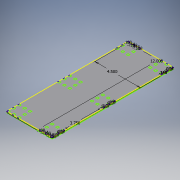
# Autodesk Inventor part: Part1
Saved by Autodesk Inventor 2018 (Build 220112000, 112)
## iProperties
Created: 2018-04-10
Part Number: Part1
Material: Generic
Document SubType Name: Modeling
Designer: Administrator
Density: 1 g/cm^3
Appearance: Default
Author: Administrator
Autodesk Inventor part; units mm, degrees
ref_plane "YZ Plane" through (0, 0, 0) normal (1, 0, 0) x (0, 1, 0)
ref_plane "XZ Plane" through (0, 0, 0) normal (0, 1, 0) x (-1, 0, 0)
ref_plane "XY Plane" through (0, 0, 0) normal (0, 0, 1) x (1, 0, 0)
sketch "Sketch1" plane through (0, 0, 0) normal (0, 1, 0) x (-1, 0, 0)
  line L0 (75.1783, 185.4548) -> (-39.1217, 185.4548)
  line L1 (-39.1217, 185.4548) -> (-39.1217, -119.3452)
  line L2 (-39.1217, -119.3452) -> (75.1783, -119.3452)
  line L3 (75.1783, -119.3452) -> (75.1783, 185.4548)
  point P0 (0, 0)
  dimension "d0" = 304.8
  dimension "d1" = 114.3
  constraints: 8 end point, 2 parallel, 1 horizontal, 1 perpendicular
  measures "d0" distance of L2.end L0.start
  measures "d1" distance of L1.end L2.end
extrude "Extrusion4" add sketch "Sketch1" along normal blind 3
sketch "Sketch11" plane through (0, 3, 0) normal (0, 1, 0) x (1, 0, 0)
  line L0 (39.1217, -185.4548) -> (34.3592, -185.4548)
  line L1 (34.3592, -185.4548) -> (34.3592, -180.6923)
  line L2 (34.3592, -180.6923) -> (39.1217, -180.6923)
  line L3 (39.1217, -180.6923) -> (39.1217, -185.4548)
  line L4 (39.1217, -185.4548) -> (39.1217, 119.3452) projected
  line L5 (39.1217, 119.3452) -> (-75.1783, 119.3452) projected
  line L6 (-75.1783, -185.4548) -> (39.1217, -185.4548) projected
  line L7 (25.628, -185.4548) -> (20.8655, -185.4548)
  line L8 (20.8655, -185.4548) -> (20.8655, -180.6923)
  line L9 (20.8655, -180.6923) -> (25.628, -180.6923)
  line L10 (25.628, -180.6923) -> (25.628, -185.4548)
  line L11 (12.1342, -185.4548) -> (7.3717, -185.4548)
  line L12 (7.3717, -185.4548) -> (7.3717, -180.6923)
  line L13 (7.3717, -180.6923) -> (12.1342, -180.6923)
  line L14 (12.1342, -180.6923) -> (12.1342, -185.4548)
  line L15 (39.1217, -171.961) -> (34.3592, -171.961)
  line L16 (34.3592, -171.961) -> (34.3592, -167.1985)
  line L17 (34.3592, -167.1985) -> (39.1217, -167.1985)
  line L18 (39.1217, -167.1985) -> (39.1217, -171.961)
  line L19 (39.1217, -158.4673) -> (34.3592, -158.4673)
  line L20 (34.3592, -158.4673) -> (34.3592, -153.7048)
  line L21 (34.3592, -153.7048) -> (39.1217, -153.7048)
  line L22 (39.1217, -153.7048) -> (39.1217, -158.4673)
  line L23 (25.628, -158.4673) -> (20.8655, -158.4673)
  line L24 (20.8655, -158.4673) -> (20.8655, -153.7048)
  line L25 (20.8655, -153.7048) -> (25.628, -153.7048)
  line L26 (25.628, -153.7048) -> (25.628, -158.4673)
  line L27 (12.1342, -158.4673) -> (7.3717, -158.4673)
  line L28 (7.3717, -158.4673) -> (7.3717, -153.7048)
  line L29 (7.3717, -153.7048) -> (12.1342, -153.7048)
  line L30 (12.1342, -153.7048) -> (12.1342, -158.4673)
  line L31 (12.1342, -171.961) -> (7.3717, -171.961)
  line L32 (7.3717, -171.961) -> (7.3717, -167.1985)
  line L33 (7.3717, -167.1985) -> (12.1342, -167.1985)
  line L34 (12.1342, -167.1985) -> (12.1342, -171.961)
  line L35 (39.1217, -58.4548) -> (34.3592, -58.4548)
  line L36 (34.3592, -58.4548) -> (34.3592, -53.6923)
  line L37 (34.3592, -53.6923) -> (39.1217, -53.6923)
  line L38 (39.1217, -53.6923) -> (39.1217, -58.4548)
  line L39 (39.1217, -44.961) -> (34.3592, -44.961)
  line L40 (34.3592, -44.961) -> (34.3592, -40.1985)
  line L41 (34.3592, -40.1985) -> (39.1217, -40.1985)
  line L42 (39.1217, -40.1985) -> (39.1217, -44.961)
  line L43 (39.1217, -31.4673) -> (34.3592, -31.4673)
  line L44 (34.3592, -31.4673) -> (34.3592, -26.7048)
  line L45 (34.3592, -26.7048) -> (39.1217, -26.7048)
  line L46 (39.1217, -26.7048) -> (39.1217, -31.4673)
  line L47 (25.628, -58.4548) -> (20.8655, -58.4548)
  line L48 (20.8655, -58.4548) -> (20.8655, -53.6923)
  line L49 (20.8655, -53.6923) -> (25.628, -53.6923)
  line L50 (25.628, -53.6923) -> (25.628, -58.4548)
  line L51 (12.1342, -58.4548) -> (7.3717, -58.4548)
  line L52 (7.3717, -58.4548) -> (7.3717, -53.6923)
  line L53 (7.3717, -53.6923) -> (12.1342, -53.6923)
  line L54 (12.1342, -53.6923) -> (12.1342, -58.4548)
  line L55 (12.1342, -44.961) -> (7.3717, -44.961)
  line L56 (7.3717, -44.961) -> (7.3717, -40.1985)
  line L57 (7.3717, -40.1985) -> (12.1342, -40.1985)
  line L58 (12.1342, -40.1985) -> (12.1342, -44.961)
  line L59 (12.1342, -31.4673) -> (7.3717, -31.4673)
  line L60 (7.3717, -31.4673) -> (7.3717, -26.7048)
  line L61 (7.3717, -26.7048) -> (12.1342, -26.7048)
  line L62 (12.1342, -26.7048) -> (12.1342, -31.4673)
  line L63 (25.628, -31.4673) -> (20.8655, -31.4673)
  line L64 (20.8655, -31.4673) -> (20.8655, -26.7048)
  line L65 (20.8655, -26.7048) -> (25.628, -26.7048)
  line L66 (25.628, -26.7048) -> (25.628, -31.4673)
  line L67 (39.1217, 119.3452) -> (34.3592, 119.3452)
  line L68 (34.3592, 119.3452) -> (34.3592, 114.5827)
  line L69 (34.3592, 114.5827) -> (39.1217, 114.5827)
  line L70 (39.1217, 114.5827) -> (39.1217, 119.3452)
  line L71 (39.1217, 105.8515) -> (34.3592, 105.8515)
  line L72 (34.3592, 105.8515) -> (34.3592, 101.089)
  line L73 (34.3592, 101.089) -> (39.1217, 101.089)
  line L74 (39.1217, 101.089) -> (39.1217, 105.8515)
  line L75 (39.1217, 92.3577) -> (34.3592, 92.3577)
  line L76 (34.3592, 92.3577) -> (34.3592, 87.5952)
  line L77 (34.3592, 87.5952) -> (39.1217, 87.5952)
  line L78 (39.1217, 87.5952) -> (39.1217, 92.3577)
  line L79 (25.628, 87.5952) -> (20.8655, 87.5952)
  line L80 (20.8655, 87.5952) -> (20.8655, 92.3577)
  line L81 (20.8655, 92.3577) -> (25.628, 92.3577)
  line L82 (25.628, 92.3577) -> (25.628, 87.5952)
  line L83 (12.1342, 87.5952) -> (7.3717, 87.5952)
  line L84 (7.3717, 87.5952) -> (7.3717, 92.3577)
  line L85 (7.3717, 92.3577) -> (12.1342, 92.3577)
  line L86 (12.1342, 92.3577) -> (12.1342, 87.5952)
  line L87 (12.1342, 101.089) -> (7.3717, 101.089)
  line L88 (7.3717, 101.089) -> (7.3717, 105.8515)
  line L89 (7.3717, 105.8515) -> (12.1342, 105.8515)
  line L90 (12.1342, 105.8515) -> (12.1342, 101.089)
  line L91 (12.1342, 114.5827) -> (7.3717, 114.5827)
  line L92 (7.3717, 114.5827) -> (7.3717, 119.3452)
  line L93 (7.3717, 119.3452) -> (12.1342, 119.3452)
  line L94 (12.1342, 119.3452) -> (12.1342, 114.5827)
  line L95 (25.628, 114.5827) -> (20.8655, 114.5827)
  line L96 (20.8655, 114.5827) -> (20.8655, 119.3452)
  line L97 (20.8655, 119.3452) -> (25.628, 119.3452)
  line L98 (25.628, 119.3452) -> (25.628, 114.5827)
  line L99 (-75.1783, 119.3452) -> (-70.4158, 119.3452)
  line L100 (-70.4158, 119.3452) -> (-70.4158, 114.5827)
  line L101 (-70.4158, 114.5827) -> (-75.1783, 114.5827)
  line L102 (-75.1783, 114.5827) -> (-75.1783, 119.3452)
  line L103 (-61.6845, 114.5827) -> (-56.922, 114.5827)
  line L104 (-56.922, 114.5827) -> (-56.922, 119.3452)
  line L105 (-56.922, 119.3452) -> (-61.6845, 119.3452)
  line L106 (-61.6845, 119.3452) -> (-61.6845, 114.5827)
  line L107 (-48.1908, 114.5827) -> (-43.4283, 114.5827)
  line L108 (-43.4283, 114.5827) -> (-43.4283, 119.3452)
  line L109 (-43.4283, 119.3452) -> (-48.1908, 119.3452)
  line L110 (-48.1908, 119.3452) -> (-48.1908, 114.5827)
  line L111 (-43.4283, 105.8515) -> (-48.1908, 105.8515)
  line L112 (-48.1908, 105.8515) -> (-48.1908, 101.089)
  line L113 (-48.1908, 101.089) -> (-43.4283, 101.089)
  line L114 (-43.4283, 101.089) -> (-43.4283, 105.8515)
  line L115 (-75.1783, 119.3452) -> (-75.1783, -185.4548) projected
  line L116 (-70.4158, 105.8515) -> (-75.1783, 105.8515)
  line L117 (-75.1783, 105.8515) -> (-75.1783, 101.089)
  line L118 (-75.1783, 101.089) -> (-70.4158, 101.089)
  line L119 (-70.4158, 101.089) -> (-70.4158, 105.8515)
  line L120 (-43.4283, 92.3577) -> (-48.1908, 92.3577)
  line L121 (-48.1908, 92.3577) -> (-48.1908, 87.5952)
  line L122 (-48.1908, 87.5952) -> (-43.4283, 87.5952)
  line L123 (-43.4283, 87.5952) -> (-43.4283, 92.3577)
  line L124 (-70.4158, 92.3577) -> (-75.1783, 92.3577)
  line L125 (-75.1783, 92.3577) -> (-75.1783, 87.5952)
  line L126 (-75.1783, 87.5952) -> (-70.4158, 87.5952)
  line L127 (-70.4158, 87.5952) -> (-70.4158, 92.3577)
  line L128 (-56.922, 92.3577) -> (-61.6845, 92.3577)
  line L129 (-61.6845, 92.3577) -> (-61.6845, 87.5952)
  line L130 (-61.6845, 87.5952) -> (-56.922, 87.5952)
  line L131 (-56.922, 87.5952) -> (-56.922, 92.3577)
  line L132 (-43.4283, -26.7048) -> (-48.1908, -26.7048)
  line L133 (-48.1908, -26.7048) -> (-48.1908, -31.4673)
  line L134 (-48.1908, -31.4673) -> (-43.4283, -31.4673)
  line L135 (-43.4283, -31.4673) -> (-43.4283, -26.7048)
  line L136 (-56.922, -26.7048) -> (-61.6845, -26.7048)
  line L137 (-61.6845, -26.7048) -> (-61.6845, -31.4673)
  line L138 (-61.6845, -31.4673) -> (-56.922, -31.4673)
  line L139 (-56.922, -31.4673) -> (-56.922, -26.7048)
  line L140 (-70.4158, -26.7048) -> (-75.1783, -26.7048)
  line L141 (-75.1783, -26.7048) -> (-75.1783, -31.4673)
  line L142 (-75.1783, -31.4673) -> (-70.4158, -31.4673)
  line L143 (-70.4158, -31.4673) -> (-70.4158, -26.7048)
  line L144 (-43.4283, -40.1985) -> (-48.1908, -40.1985)
  line L145 (-48.1908, -40.1985) -> (-48.1908, -44.961)
  line L146 (-48.1908, -44.961) -> (-43.4283, -44.961)
  line L147 (-43.4283, -44.961) -> (-43.4283, -40.1985)
  line L148 (-43.4283, -53.6923) -> (-48.1908, -53.6923)
  line L149 (-48.1908, -53.6923) -> (-48.1908, -58.4548)
  line L150 (-48.1908, -58.4548) -> (-43.4283, -58.4548)
  line L151 (-43.4283, -58.4548) -> (-43.4283, -53.6923)
  line L152 (-56.922, -53.6923) -> (-61.6845, -53.6923)
  line L153 (-61.6845, -53.6923) -> (-61.6845, -58.4548)
  line L154 (-61.6845, -58.4548) -> (-56.922, -58.4548)
  line L155 (-56.922, -58.4548) -> (-56.922, -53.6923)
  line L156 (-70.4158, -53.6923) -> (-75.1783, -53.6923)
  line L157 (-75.1783, -53.6923) -> (-75.1783, -58.4548)
  line L158 (-75.1783, -58.4548) -> (-70.4158, -58.4548)
  line L159 (-70.4158, -58.4548) -> (-70.4158, -53.6923)
  line L160 (-70.4158, -40.1985) -> (-75.1783, -40.1985)
  line L161 (-75.1783, -40.1985) -> (-75.1783, -44.961)
  line L162 (-75.1783, -44.961) -> (-70.4158, -44.961)
  line L163 (-70.4158, -44.961) -> (-70.4158, -40.1985)
  line L164 (-43.4283, -153.7048) -> (-48.1908, -153.7048)
  line L165 (-48.1908, -153.7048) -> (-48.1908, -158.4673)
  line L166 (-48.1908, -158.4673) -> (-43.4283, -158.4673)
  line L167 (-43.4283, -158.4673) -> (-43.4283, -153.7048)
  line L168 (-56.922, -153.7048) -> (-61.6845, -153.7048)
  line L169 (-61.6845, -153.7048) -> (-61.6845, -158.4673)
  line L170 (-61.6845, -158.4673) -> (-56.922, -158.4673)
  line L171 (-56.922, -158.4673) -> (-56.922, -153.7048)
  line L172 (-70.4158, -153.7048) -> (-75.1783, -153.7048)
  line L173 (-75.1783, -153.7048) -> (-75.1783, -158.4673)
  line L174 (-75.1783, -158.4673) -> (-70.4158, -158.4673)
  line L175 (-70.4158, -158.4673) -> (-70.4158, -153.7048)
  line L176 (-43.4283, -167.1985) -> (-48.1908, -167.1985)
  line L177 (-48.1908, -167.1985) -> (-48.1908, -171.961)
  line L178 (-48.1908, -171.961) -> (-43.4283, -171.961)
  line L179 (-43.4283, -171.961) -> (-43.4283, -167.1985)
  line L180 (-43.4283, -180.6923) -> (-48.1908, -180.6923)
  line L181 (-48.1908, -180.6923) -> (-48.1908, -185.4548)
  line L182 (-48.1908, -185.4548) -> (-43.4283, -185.4548)
  line L183 (-43.4283, -185.4548) -> (-43.4283, -180.6923)
  line L184 (-56.922, -180.6923) -> (-61.6845, -180.6923)
  line L185 (-61.6845, -180.6923) -> (-61.6845, -185.4548)
  line L186 (-61.6845, -185.4548) -> (-56.922, -185.4548)
  line L187 (-56.922, -185.4548) -> (-56.922, -180.6923)
  line L188 (-70.4158, -180.6923) -> (-75.1783, -180.6923)
  line L189 (-75.1783, -180.6923) -> (-75.1783, -185.4548)
  line L190 (-75.1783, -185.4548) -> (-70.4158, -185.4548)
  line L191 (-70.4158, -185.4548) -> (-70.4158, -180.6923)
  line L192 (-70.4158, -171.961) -> (-75.1783, -171.961)
  line L193 (-75.1783, -171.961) -> (-75.1783, -167.1985)
  line L194 (-75.1783, -167.1985) -> (-70.4158, -167.1985)
  line L195 (-70.4158, -167.1985) -> (-70.4158, -171.961)
  dimension "d169" = 4.7625
  dimension "d229" = 4.7625
  dimension "d230" = 4.7625
  dimension "d231" = 8.7312
  dimension "d232" = 8.7312
  dimension "d233" = 4.7625
  dimension "d234" = 8.7312
  dimension "d235" = 4.7625
  dimension "d236" = 4.7625
  dimension "d237" = 8.7312
  dimension "d238" = 4.7625
  dimension "d239" = 95.25
  dimension "d240" = 8.7312
  dimension "d241" = 4.7625
  dimension "d242" = 4.7625
  dimension "d243" = 8.7312
  dimension "d244" = 4.7625
  dimension "d245" = 8.7312
  dimension "d246" = 4.7625
  dimension "d247" = 4.7625
  dimension "d248" = 8.7312
  dimension "d249" = 4.7625
  dimension "d250" = 8.7312
  dimension "d251" = 4.7625
  dimension "d252" = 4.7625
  dimension "d253" = 8.7312
  constraints: 384 end point, 96 parallel, 74 point on line, 48 horizontal, 48 perpendicular, 16 other
  measures "d169" distance between parallel lines of L3 L1
  measures "d229" distance between parallel lines of L2 L0
  measures "d230" distance between parallel lines of L8 L10
  measures "d231" distance between parallel lines of L1 L10
  measures "d232" distance between parallel lines of L8 L14
  measures "d233" distance between parallel lines of L12 L14
  measures "d234" distance between parallel lines of L2 L15
  measures "d235" distance between parallel lines of L17 L15
  measures "d236" distance between parallel lines of L19 L21
  measures "d237" distance between parallel lines of L17 L19
  measures "d238" distance between parallel lines of L37 L35
  measures "d239" distance between parallel lines of L21 L35
  measures "d240" distance between parallel lines of L39 L37
  measures "d241" distance between parallel lines of L41 L39
  measures "d242" distance between parallel lines of L45 L43
  measures "d243" distance between parallel lines of L41 L43
  measures "d244" distance between parallel lines of L71 L73
  measures "d245" distance between parallel lines of L69 L71
  measures "d246" distance between parallel lines of L5 L69
  measures "d247" distance between parallel lines of L75 L77
  measures "d248" distance between parallel lines of L73 L75
  measures "d249" distance between parallel lines of L102 L100
  measures "d250" distance between parallel lines of L100 L106
  measures "d251" distance between parallel lines of L104 L106
  measures "d252" distance between parallel lines of L108 L110
  measures "d253" distance between parallel lines of L104 L110
body "Solid1"
